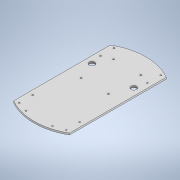
# Autodesk Inventor part: basePlate3
Saved by Autodesk Inventor 2020 (Build 240168000, 168)
## iProperties
Created: 2020-02-05
Part Number: basePlate3
Material: Generic
Document SubType Name: Modeling
Designer: mdjb501
Density: 1 g/cm^3
Appearance: Default
Author: mdjb501
Autodesk Inventor part; units mm, degrees
ref_plane "YZ Plane" through (0, 0, 0) normal (1, 0, 0) x (0, 1, 0)
ref_plane "XZ Plane" through (0, 0, 0) normal (0, 1, 0) x (-1, 0, 0)
ref_plane "XY Plane" through (0, 0, 0) normal (0, 0, 1) x (1, 0, 0)
sketch "Sketch1" plane through (0, 0, 0) normal (0, 1, 0) x (-1, 0, 0)
  line L0 (-50, 86.6025) -> (-50, -86.6025)
  line L1 (50, -86.6025) -> (50, 86.6025)
  arc A0 (50, 86.6025) -> (-50, 86.6025) centre (0, 0) ccw
  arc A1 (-50, -86.6025) -> (50, -86.6025) centre (0, 0) ccw
  circle A2 centre (25, -67.0117) radius 1.35
  circle A3 centre (25, -9.0117) radius 1.35
  circle A4 centre (-24, -9.0117) radius 1.35
  circle A5 centre (-24, -67.0117) radius 1.35
  circle A6 centre (42, -84.8528) radius 1.3
  circle A7 centre (42, -60.6528) radius 1.3
  circle A8 centre (-42, -84.8528) radius 1.3
  circle A9 centre (-42, -60.6528) radius 1.3
  circle A10 centre (42, 84.8528) radius 1.3
  circle A11 centre (42, 60.6528) radius 1.3
  circle A12 centre (-42, 84.8528) radius 1.3
  circle A13 centre (-42, 60.6528) radius 1.3
  circle A14 centre (23.5943, 91.1005) radius 1.3
  circle A15 centre (-23.9057, 91.1005) radius 1.3
  circle A16 centre (37.5, -41.0117) radius 5
  circle A17 centre (-37.5, -41.0117) radius 5
  constraints: 18 centre point, 4 end point, 4 point on circle, 1 coincident, 1 parallel
extrude "Extrusion1" add sketch "Sketch1" along normal blind 3
body "Solid1"
